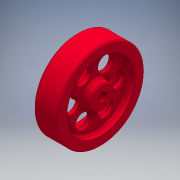
# Autodesk Inventor part: flywheel
Saved by Autodesk Inventor 2017 (Build 210142000, 142)
## iProperties
Created: 2018-11-17
Part Number: flywheel
Material: Iron, Cast
Document SubType Name: Modeling
Designer: Arman Grewal
Density: 7.15 g/cm^3
Appearance: Iron Gray
Author: Arman Grewal
Autodesk Inventor part; units mm, degrees
ref_plane "YZ Plane" through (0, 0, 0) normal (1, 0, 0) x (0, 1, 0)
ref_plane "XZ Plane" through (0, 0, 0) normal (0, 1, 0) x (-1, 0, 0)
ref_plane "XY Plane" through (0, 0, 0) normal (0, 0, 1) x (1, 0, 0)
sketch "Sketch1" plane through (0, 0, 0) normal (1, 0, 0) x (0, 1, 0)
  circle A0 centre (0, 0) radius 41
  dimension "d0" = 82
  constraints: 1 centre point, 1 coincident
  measures "d0" diameter of A0
extrude "Extrusion1" add sketch "Sketch1" along normal blind 22
sketch "Sketch2" plane through (22, 0, 0) normal (1, 0, 0) x (0, 0, -1)
  circle A0 centre (0, 0) radius 11
  circle A1 centre (0, 0) radius 32
  dimension "d3" = 22
  dimension "d4" = 64
  constraints: 2 centre point, 2 coincident
  measures "d3" diameter of A0
  measures "d4" diameter of A1
extrude "Extrusion2" cut sketch "Sketch2" against normal blind 6
sketch "Sketch3" plane through (22, 0, 0) normal (1, 0, 0) x (0, 0, -1)
  circle A0 centre (0, 0) radius 11
  dimension "d7" = 22
  constraints: 1 centre point, 1 coincident
  measures "d7" diameter of A0
extrude "Extrusion3" add sketch "Sketch3" along normal blind 1.5
sketch "Sketch4" plane through (23.5, 0, 0) normal (1, 0, 0) x (0, 0, -1)
  circle A0 centre (0, 0) radius 4
  dimension "d10" = 8
  constraints: 1 centre point, 1 coincident
  measures "d10" diameter of A0
extrude "Extrusion4" cut sketch "Sketch4" against normal blind 23.5
sketch "Sketch5" plane through (0, 0, 0) normal (-1, 0, 0) x (0, 0, 1)
  circle A0 centre (0, 0) radius 11
  circle A1 centre (0, 0) radius 4
  dimension "d13" = 22
  dimension "d14" = 8
  constraints: 2 centre point, 2 coincident
  measures "d13" diameter of A0
  measures "d14" diameter of A1
extrude "Extrusion5" cut sketch "Sketch5" against normal blind 1.5
sketch "Sketch6" plane through (0, 0, 0) normal (-1, 0, 0) x (0, 0, 1)
  circle A0 centre (0, 0) radius 11
  circle A1 centre (0, 0) radius 32
  dimension "d17" = 64
  dimension "d18" = 22
  constraints: 2 centre point, 2 coincident
  measures "d17" diameter of A1
  measures "d18" diameter of A0
extrude "Extrusion6" cut sketch "Sketch6" against normal blind 12
chamfer "Chamfer1" distance 1 angle 45 4 edges at (22, -41, 0) (0, -41, 0) (23.5, 0, 11) (1.5, 0, -11)
sketch "Sketch7" plane through (12, 0, 0) normal (-1, 0, 0) x (0, 0, 1)
  circle A0 centre (0, 0) radius 21 construction
  circle A1 centre (0, 21) radius 7
  circle A2 centre (-18.1865, 10.5) radius 7
  circle A3 centre (-18.1865, -10.5) radius 7
  circle A4 centre (0, -21) radius 7
  circle A5 centre (18.1865, -10.5) radius 7
  circle A6 centre (18.1865, 10.5) radius 7
  dimension "d24" = 42
  dimension "d25" = 14
  dimension "d28" = 360
  dimension "d30" = 10.5
  constraints: 6 centre point, 1 coincident, 1 vertical alignment, 15 other
  measures "d25" diameter of A1
  measures "d30" vertical distance of A6.centre A1.centre
extrude "Extrusion7" cut sketch "Sketch7" against normal up to next
chamfer "Chamfer2" distance 0.5 angle 45 7 edges at (16, 21, -7) (12, 21, -7) (16, 10.5, -25.1865) (12, 10.5, -25.1865) (16, -10.5, -25.1865) (12, -10.5, -25.1865) (16, 10.5, 11.1865)
chamfer "Chamfer3" distance 0.5 angle 45 4 edges at (16, -10.5, 11.1865) (12, -10.5, 11.1865) (16, -21, -7) (12, -21, -7)
fillet "Fillet1" radius 2 4 edges at (12, 0, -11) (12, 0, -32) (16, 0, 32) (16, 0, 11)
sketch "Sketch8" plane through (0, 0, 0) normal (0, 1, 0) x (-1, 0, 0)
  line L0 (0, 0) -> (-2.5, 0) construction
  line L1 (-2.5, -11) -> (-2.5, 11) projected
  line L2 (-2.5, 0) -> (-6.5, 0) construction
  circle A0 centre (-6.5, 0) radius 1.5
  dimension "d40" = 4
  dimension "d41" = 3
  constraints: 4 end point, 1 centre point, 1 coincident, 1 horizontal, 1 midpoint
  measures "d40" distance of L0.end L2.end
  measures "d41" diameter of A0
extrude "Extrusion8" cut sketch "Sketch8" along normal blind 12
thread "Thread1" size "M3x0.5" class "6H" standard "ANSI Metric M Profile" full length
body "Solid1"
